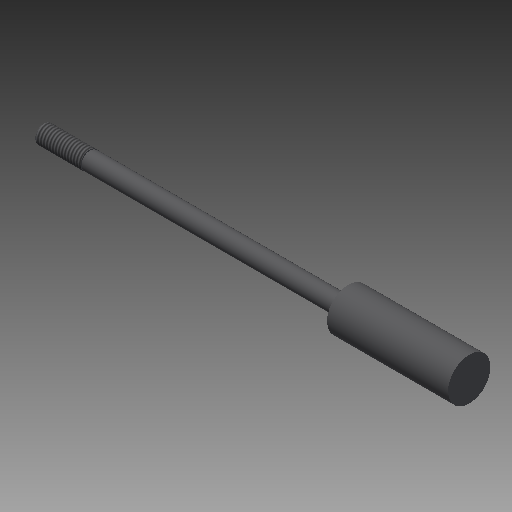
# Autodesk Inventor part: M-011-BT1EE110_rod
Saved by Autodesk Inventor 2017 (Build 210142000, 142)
## iProperties
Category: PARTsolutions
Company: BIMBA
Created: 2017-01-31
Part Number: M-011-BT1EE110_rod
Catalog Web Link: www.cadenas.de
Description: Standard Air Cylinder_rod-Original Line - Standard Air Cylinders
Vendor: BIMBA
Document SubType Name: Modeling
Designer: psAdmin
Manufacturer: BIMBA
Mass: 4.62498 g
Surface Area: 25.4583 cm^2
Volume: 4.62498 cm^3
Density: 1 g/cm^3
Material: Generic
Appearance: PSOLRGB-181-181-181
PSOL_IDENT_0: {$CADENAS_DATA\23d-libs\bimba\bimba\bimba_imperial\bimba_full_line\original_line_cylinders\standard_
PSOL_IDENT_1: air_cylinders\rod.prj},302 {VTYP=3D},{NB=M-011-BT1EE110_rod},{LINA=M-011-BT1EE110_rod},{NN=Standard
PSOL_IDENT_2: Air Cylinder_rod},{DATE=09.11.2016 07:55:11},{GEOMDATE=10.09.2015 10:40:00},{VERSION=},{LINEID=30},{
PSOL_IDENT_3: LINESUBID=-1},{WBVAR=STROKE,ACTING,MNT,DER,NR,BM,CO,M,EE,EEL,K,Q,Y,F,G,T,B,H,SER,SR,NT,W,E,HL,ST,STP
PSOL_IDENT_4: ,PRC,PB,COLOR1,FCD,RCD,BCD}  {NB=M-011-BT1EE110_rod},{LINA=M-011-BT1EE110_rod},{KT=DUMMY},{PN=M-011-
PSOL_IDENT_5: BT1EE11},{DASH=-},{BORE=0.43750000},{BOREPN=01},{STROKE=1.000},{STROKEALG=[0.001:50/0.001]},{STROKE1=
PSOL_IDENT_6: 1.000},{ACTING=},{ACTINGALG= '' , 'Single Acting' , 'R' , 'Reverse Single Acting' , 'D' , 'Double Ac
PSOL_IDENT_7: ting' },{ACTINGPN=},{MNT=},{MNTALG= '' , 'Front Nose Mounting' , 'P' , 'Rear Pivot Mounting' , 'BF'
PSOL_IDENT_8: , 'Front Block Mounting' , 'BR' , 'Rear Block Mounting for Vertical Positioning' , 'BFT' , 'Front Bl
PSOL_IDENT_9: ock Trunnion Mounting' , 'BRT' , 'Rear Block Trunnion Mounting' },{TYPE=M-},{MNTPN=},{DER=},{DERALG=
PSOL_IDENT_10: '' , 'N/A' },{NR=},{NRALG= '' , 'Standard' , 'NR' , 'Non-rotating - Hexagon Rod' },{NRPN=},{BM=},{B
PSOL_IDENT_11: MALG= '' , 'N/A' },{BMPN=},{CO=},{COALG= '' , 'N/A' },{M=M},{MALG= '', 'Without Magnet', 'M', 'With
PSOL_IDENT_12: Magnet' },{EE=EE},{EEL=1},{EEMAX=49},{EEALG= '', 'Without Extra Extension', 'EE', 'With Extra Extens
PSOL_IDENT_13: ion' },{EELALG=[0.001:49/0.001]},{EEPN=EE1},{EEPN1=1.000},{K=},{KALG= '' , 'N/A' },{KPN=},{Q=},{QALG=
PSOL_IDENT_14: '' , 'Without Side Ported Rear Head' , 'Q' , 'With Side Ported Rear Head' },{QPN=},{Y=},{YALG= '' ,
PSOL_IDENT_15: 'N/A' },{YPN=},{F=},{FALG= '', 'Standard', 'F', 'Molycoated Body' },{FPN=},{G=},{GPN=},{T=},{TALG= ''
PSOL_IDENT_16: , 'Standard' , 'N' , 'Low Temperature' , 'V' , 'High Temperature' },{NPN=},{VPN=},{B=B},{BALG= '', '
PSOL_IDENT_17: Without Bumper' , 'B' , 'With Bumper' },{BPN=B},{H=},{HALG= '', 'N/A' },{HPN=},{SER=},{SERALG= '' , '
PSOL_IDENT_18: N/A' },{SR=},{SRALG= 'C' , 'Carbon Steel Rod' , 'SR' , '303 Stainless Steel Rod' , '' , '303 Stainle
PSOL_IDENT_19: ss Steel Rod1' },{SRPN=},{SRCON=0},{NT=},{NTPN=},{W=},{WALG= '' , 'N/A' },{WPN=},{E=},{EALG= '' , 'W
PSOL_IDENT_20: ithout Special Lube and Seals' , 'E' , 'With Special Lube and Seals' },{EPN=},{HL=},{HLALG= '' , 'N/
PSOL_IDENT_21: A' },{ST=T},{STALG= 'T' , 'With Switch Track' },{STP=1},{STPALG= '1' , 'T1' , '2' , 'T2' , '3' , 'T3'
PSOL_IDENT_22: , '4' , 'T4' },{STPN=T1},{PRC=},{PRCALG= '' , 'Without Piston Rod Clevis' , 'D-166-1' , 'With Pisto
PSOL_IDENT_23: n Rod Clevis' },{PRCPN=},{PB=},{PBALG= '' , 'Without Pivot Bracket' , 'D-167' , 'With Pivot Bracket'
PSOL_IDENT_24: },{PBPN=},{TLEN=2.6620},{TEXT=0.166667},{SPACE=0.095238},{FRAC=3.1900},{RGCON=},{RGDACCON=},{RHCON=
PSOL_IDENT_25: },{RHCONON=1},{RHACCON=},{FNUTCON=1},{RNUTCON=0},{FNUTPN=D-801},{RNUTPN=},{FNUTTRANS=0.0000},{RNUTTR
PSOL_IDENT_26: ANS=0.0000},{VHOLECON=2},{A1=0.6880},{A1N=0.6880},{A1P=1.1880},{A1B=1.1880},{A4=0.2500},{A4N=0.2500}
PSOL_IDENT_27: ,{A4P=0.1880},{A5=0.0200},{A1H=0.5},{A1NH=0.5000},{A1PH=1.1880},{A1BH=0.8120},{A1SH=0.0000},{A2H=0.1
PSOL_IDENT_28: 880},{A2NH=0.1880},{LENGTH=1.3100},{LENGTH1=1.3100},{LENGTH2=2.1700},{MUL=1.8800},{MUL11=1.8800},{MU
PSOL_IDENT_29: L22=2.8800},{MUL33=1.8800},{MUL2=0.9400},{MUL211=0.9400},{MUL222=1.4400},{MUL233=0.9400},{SSS=2.0000
PSOL_IDENT_30: },{RGLEN=0.4580},{RHLEN=0.3320},{SSS1=2.0000},{A13=0.9380},{THDLEN1=0.5000},{THD1=0.1900},{TAB=UNF},
PSOL_IDENT_31: {THDLEN=0.5000},{THD=0.1900},{OD=0.4465},{RODL=3.4520},{PL=1.2640},{RODDIA=0.1870},{HEX=0.1870},{ROD
PSOL_IDENT_32: TRANS=1.0000},{G1=0.0000},{ON=0},{G5=0.0000},{DERLEN=2.1880},{THOLE=0.0000},{WF=0.0000},{BADD=0.0620
PSOL_IDENT_33: },{MADD=0.2000},{NVADD=0.000},{JRADD=0.00000},{COLOR=0.71,0.71,0.71,0.00},{GROOVE=1},{HOL=0},{D7=0.1
PSOL_IDENT_34: 590},{H1=0.0000},{D1=0.4840},{D1RH=0.4855},{D1P=0.0000},{D1B=0.7380},{D1N=0.4840},{D1NRH=0.4855},{D1
PSOL_IDENT_35: BRH=0.4855},{D1PRH=0.7380},{BOZO=0},{HADD=0.000},{COLOR1=0},{DEFL=0.0000},{HEXL=0.0000},{SSADD=0.000
PSOL_IDENT_36: 0},{WFL=0.0000},{MOVE=0.0000},{PRCL2=0.37500},{PRCB=0.12000},{PRCTRANS=0.00000},{FCD=0},{RCD=0},{BCD=
PSOL_IDENT_37: 0}
NN: Standard Air Cylinder_rod
NT: Standard
NB: M-011-BT1EE110_rod
NBSYN: $PN.$COLOR1._rod
LINA: M-011-BT1EE110_rod
PN: M-011-BT1EE11
BORE: 0.43750000
BOREPN: 01
STROKE: 1.000
ACTING: Single Acting
MNT: Front Nose Mounting
DER: N/A
NR: Standard
BM: N/A
CO: N/A
M: With Magnet
EE: With Extra Extension
EEL: 1
K: N/A
Q: Without Side Ported Rear Head
Y: N/A
F: Standard
G: Without Magnalube Lubrication
T: Standard
B: With Bumper
H: N/A
SER: N/A
SR: 303 Stainless Steel Rod1
W: N/A
E: Without Special Lube and Seals
HL: N/A
ST: With Switch Track
STP: T1
PRC: Without Piston Rod Clevis
PB: Without Pivot Bracket
A1N: 0.6880
A1P: 1.1880
A1B: 1.1880
A4N: 0.2500
A4P: 0.1880
A5: 0.0200
A1NH: 0.5000
A1PH: 1.1880
A1BH: 0.8120
A1SH: 0.0000
A2NH: 0.1880
A13: 0.9380
THDLEN1: 0.5000
THD1: 0.1900
TAB: UNF
OD: 0.4465
RODDIA: 0.1870
HEX: 0.1870
G1: 0.0000
G5: 0.0000
THOLE: 0.0000
WF: 0.0000
GROOVE: 1
D7: 0.1590
D1P: 0.0000
D1B: 0.7380
D1N: 0.4840
D1NRH: 0.4855
D1BRH: 0.4855
D1PRH: 0.7380
COLOR1: 0
FCD: 0
RCD: 0
BCD: 0
SUPPLIER: BIMBA
ARTICLENO: M-011-BT1EE110_rod
BOMINFO: M-011-BT1EE110_rod
CREATOR: CADENAS GmbH
Title: M-011-BT1EE110_rod
Author: Cadenas PARTsolutions
Comments: Original Line - Standard Air Cylinders
Autodesk Inventor part; units mm, degrees
sketch "Sketch_1" plane through (0, 0, 0) normal (0, 0, 1) x (1, 0, 0)
  line L0 (100.3808, 0) -> (0, 0)
  line L1 (0, 0) -> (0, 2.3749)
  line L2 (0, 2.3749) -> (68.2752, 2.3749)
  line L3 (68.2752, 2.3749) -> (68.2752, 5.6197)
  line L4 (68.2752, 5.6197) -> (100.3808, 5.6197)
  line L5 (100.3808, 5.6197) -> (100.3808, 0)
  line L6 (100.3808, 0) -> (0, 0)
  constraints: 14 end point
revolve "Revolution1" add sketch "Sketch_1" angle 360 about axis through (100.3808, 0, 0) along (1, 0, 0)
sketch "Sketch_3" plane through (0, 0, 0) normal (0, 0, 1) x (1, 0, 0)
  line L0 (0, 0) -> (-12.7, 0)
  line L1 (-12.7, 0) -> (-12.7, 1.9406)
  line L2 (-12.7, 1.9406) -> (-12.2276, 2.413)
  line L3 (-12.2276, 2.413) -> (0, 2.413)
  line L4 (0, 2.413) -> (0, 0)
  line L5 (0, 0) -> (-12.7, 0)
  constraints: 12 end point
revolve "Revolution2" add sketch "Sketch_3" angle 360 about axis through (0, 0, 0) along (1, 0, 0)
thread "Thread1" size "10-32 UNF" class "2A" standard "ANSI Unified Screw Threads" full length
sketch "Sketch_30" plane through (0, 0, 0) normal (0, 0, 1) x (1, 0, 0)
  line L0 (0, 0) -> (-0.254, 0)
  line L1 (-0.254, 2.159) -> (0, 2.159)
  line L2 (0, 2.159) -> (0, 2.667)
  line L3 (0, 2.667) -> (-0.254, 2.667)
  line L4 (-0.254, 2.667) -> (-0.254, 2.159)
  constraints: 10 end point
revolve "Revolution3" cut sketch "Sketch_30" angle 360 about axis through (0, 0, 0) along (1, 0, 0)
ref_plane "dia1_XY" through (0, 2.3749, 0) normal (1, 0, 0) x (0, 0, -1)
ref_plane "dia1_YZ" through (0, 2.3749, 0) normal (0, 0, -1) x (0, 1, 0)
ref_plane "dia1_ZX" through (0, 2.3749, 0) normal (0, 1, 0) x (1, 0, 0)
ref_plane "dia12_XY" through (0, 0, 6.1468) normal (1, 0, 0) x (0, 0, -1)
ref_plane "dia12_YZ" through (0, 0, 6.1468) normal (0, 0, -1) x (0, 1, 0)
ref_plane "dia12_ZX" through (0, 0, 6.1468) normal (0, 1, 0) x (1, 0, 0)
ref_plane "dia2_XY" through (0, -2.3749, 0) normal (1, 0, 0) x (0, 0, -1)
ref_plane "dia2_YZ" through (0, -2.3749, 0) normal (0, 0, -1) x (0, 1, 0)
ref_plane "dia2_ZX" through (0, -2.3749, 0) normal (0, 1, 0) x (1, 0, 0)
ref_plane "dia22_XY" through (0, 0, -6.1468) normal (1, 0, 0) x (0, 0, -1)
ref_plane "dia22_YZ" through (0, 0, -6.1468) normal (0, 0, -1) x (0, 1, 0)
ref_plane "dia22_ZX" through (0, 0, -6.1468) normal (0, 1, 0) x (1, 0, 0)
ref_plane "rl1_XY" through (-12.7, 0, 0) normal (1, 0, 0) x (0, 0, -1)
ref_plane "rl1_YZ" through (-12.7, 0, 0) normal (0, 0, -1) x (0, 1, 0)
ref_plane "rl1_ZX" through (-12.7, 0, 0) normal (0, 1, 0) x (1, 0, 0)
ref_plane "rl2_XY" through (0, 0, 0) normal (1, 0, 0) x (0, 0, -1)
ref_plane "rl2_YZ" through (0, 0, 0) normal (0, 0, -1) x (0, 1, 0)
ref_plane "rl2_ZX" through (0, 0, 0) normal (0, 1, 0) x (1, 0, 0)
ref_plane "rod_cp_XY" through (0, 0, 0) normal (1, 0, 0) x (0, 0, -1)
ref_plane "rod_cp_YZ" through (0, 0, 0) normal (0, 0, -1) x (0, 1, 0)
ref_plane "rod_cp_ZX" through (0, 0, 0) normal (0, 1, 0) x (1, 0, 0)
ref_plane "thd1_XY" through (-12.7, 2.413, 0) normal (1, 0, 0) x (0, 0, -1)
ref_plane "thd1_YZ" through (-12.7, 2.413, 0) normal (0, 0, -1) x (0, 1, 0)
ref_plane "thd1_ZX" through (-12.7, 2.413, 0) normal (0, 1, 0) x (1, 0, 0)
ref_plane "thd2_XY" through (-12.7, -2.413, 0) normal (1, 0, 0) x (0, 0, -1)
ref_plane "thd2_YZ" through (-12.7, -2.413, 0) normal (0, 0, -1) x (0, 1, 0)
ref_plane "thd2_ZX" through (-12.7, -2.413, 0) normal (0, 1, 0) x (1, 0, 0)
ref_plane "to_rod_clevis_XY" through (-12.7, 0, 0) normal (1, 0, 0) x (0, 0, -1)
ref_plane "to_rod_clevis_YZ" through (-12.7, 0, 0) normal (0, 0, -1) x (0, 1, 0)
ref_plane "to_rod_clevis_ZX" through (-12.7, 0, 0) normal (0, 1, 0) x (1, 0, 0)
body "Solid1"
